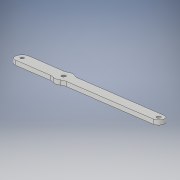
# Autodesk Inventor part: 連接7
Saved by Autodesk Inventor 2017 (Build 210142000, 142)
## iProperties
Part Number: 連接7
Material: 一般
Document SubType Name: Modeling
Designer: User
Density: 1 g/cm^3
Appearance: 預設
Author: User
Autodesk Inventor part; units mm, degrees
ref_plane "YZ Plane" through (0, 0, 0) normal (1, 0, 0) x (0, 1, 0)
ref_plane "XZ Plane" through (0, 0, 0) normal (0, 1, 0) x (-1, 0, 0)
ref_plane "XY Plane" through (0, 0, 0) normal (0, 0, 1) x (1, 0, 0)
sketch "草圖1" plane through (0, 0, 0) normal (0, 1, 0) x (-1, 0, 0)
  circle A0 centre (0, 0) radius 1.25
  circle A1 centre (-35, 0) radius 1.5
  circle A2 centre (-115, 0) radius 1.5
  arc A3 (0, -4.75) -> (0, 4.75) centre (0, 0) ccw
  arc A4 (-115, 4) -> (-115, -4) centre (-115, 0) ccw
  line L0 (0, 4.75) -> (-29.2175, 4.75)
  line L1 (-115, 4) -> (-42.2111, 4)
  line L2 (0, -4.75) -> (-29.2175, -4.75)
  line L3 (-115, -4) -> (-42.2111, -4)
  arc A5 (-32.5218, 5.4643) -> (-38.0905, 5.1429) centre (-35, 0) ccw
  arc A6 (-38.0905, -5.1429) -> (-32.5218, -5.4643) centre (-35, 0) ccw
  arc A7 (-32.5218, 5.4643) -> (-29.2175, 4.75) centre (-29.2175, 12.75) ccw
  arc A8 (-42.2111, 4) -> (-38.0905, 5.1429) centre (-42.2111, 12) ccw
  arc A9 (-38.0905, -5.1429) -> (-42.2111, -4) centre (-42.2111, -12) ccw
  arc A10 (-29.2175, -4.75) -> (-32.5218, -5.4643) centre (-29.2175, -12.75) ccw
  point P0 (-31.3343, 4.75)
  point P1 (-39.4721, 4)
  point P2 (-31.3343, -4.75)
  point P3 (-39.4721, -4)
  dimension "d0" = 2.5
  dimension "d2" = 3
  dimension "d3" = 35
  dimension "d4" = 3
  dimension "d5" = 9.5
  dimension "d6" = 8
  dimension "d8" = 8
  constraints: 20 point on circle, 11 centre point, 10 tangent, 8 end point, 4 coincident, 4 point on line, 3 equal radius
  measures "d0" diameter of A0
  measures "d2" diameter of A1
  measures "d3" distance of A0.centre A1.centre
  measures "d4" diameter of A2
  measures "d5" diameter of A3
  measures "d6" diameter of A4
  measures "d8" radius of A7
extrude "擠出1" add sketch "草圖1" along normal mid plane 3
